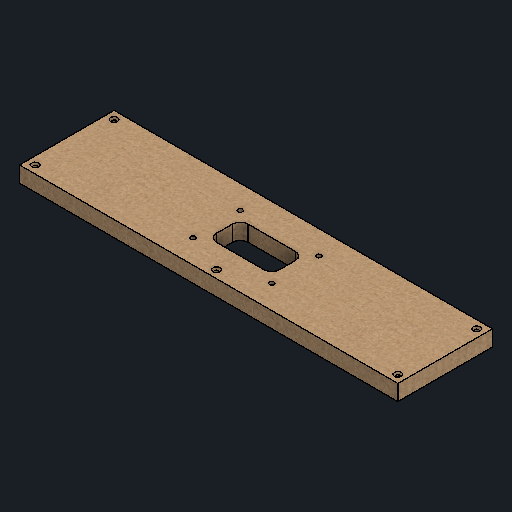
# Autodesk Inventor part: Part3
Saved by Autodesk Inventor 2026.2 (Build 302298000, 298)
## iProperties
Created: 2026-06-15
Part Number: Part3
Material: MDF Medium Density Fiberboard
Document SubType Name: Modeling
Designer: JoshuaEah
Density: 0.8 g/cm^3
Appearance: Cardboard - Corrugated
Author: JoshuaEah
Autodesk Inventor part; units mm, degrees
ref_plane "YZ Plane" through (0, 0, 0) normal (1, 0, 0) x (0, 1, 0)
ref_plane "XZ Plane" through (0, 0, 0) normal (0, 1, 0) x (-1, 0, 0)
ref_plane "XY Plane" through (0, 0, 0) normal (0, 0, 1) x (1, 0, 0)
sketch "Sketch1" plane through (0, 0, 0) normal (0, 1, 0) x (-1, 0, 0)
  line L0 (0, 0) -> (-304.8, 0)
  line L1 (-304.8, 0) -> (-304.8, -76.2)
  line L2 (-304.8, -76.2) -> (0, -76.2)
  line L3 (0, -76.2) -> (0, 0)
  line L4 (-152.4, -76.2) -> (-152.4, 0)
  line L5 (-304.8, -38.1) -> (0, -38.1)
  line L6 (-127, -50.8) -> (-177.8, -50.8)
  line L7 (-177.8, -50.8) -> (-177.8, -25.4)
  line L8 (-177.8, -25.4) -> (-127, -25.4)
  line L9 (-127, -25.4) -> (-127, -50.8)
  line L10 (-127, -50.8) -> (-177.8, -25.4) construction
  line L11 (-177.8, -50.8) -> (-127, -25.4) construction
  line L12 (-120.65, -57.15) -> (-184.15, -57.15) construction
  line L13 (-184.15, -57.15) -> (-184.15, -19.05) construction
  line L14 (-184.15, -19.05) -> (-120.65, -19.05) construction
  line L15 (-120.65, -19.05) -> (-120.65, -57.15) construction
  circle A0 centre (-120.65, -57.15) radius 1.5875
  circle A1 centre (-184.15, -57.15) radius 1.5875
  circle A2 centre (-120.65, -19.05) radius 1.5875
  circle A3 centre (-184.15, -19.05) radius 1.5875
  point P0 (-6.35, -69.85)
  point P1 (-152.4, -38.1)
  point P2 (-6.35, -69.85)
  point P3 (-298.45, -69.85)
  point P4 (-6.35, -6.35)
  point P5 (-298.45, -6.35)
  point P6 (-152.4, -6.35)
  dimension "d0" = 76.2
  dimension "d1" = 304.8
  dimension "d5" = 6.35
  dimension "d6" = 6.35
  dimension "d16" = 50.8
  dimension "d17" = 25.4
  dimension "d19" = 6.35
  dimension "d20" = 3.175
  constraints: 32 end point, 7 midpoint, 6 parallel, 6 symmetric about line, 4 centre point, 3 coincident, 3 perpendicular, 2 horizontal, 1 horizontal alignment, 1 point on line, 6 other
  measures "d0" distance of L2.end L0.start
  measures "d1" distance of L0.start L0.end
  measures "d5" distance from line of point (-6.35, -69.85) L3
  measures "d6" distance from line of L2 point (-6.35, -69.85)
  measures "d16" distance of L7.end L8.end
  measures "d17" distance of L6.end L7.end
  measures "d19" distance between parallel lines of L9 L15
  measures "d20" diameter of A0
extrude "Extrusion1" add sketch "Sketch1" against normal blind 12.7 contours L3 L5 L9 L8 L4 L0 | L4 L8 L7 L5 L1 L0 | L3 L2 L4 L6 L9 L5 | L5 L7 L6 L4 L2 L1 | A0 | A1 | A2 | A3
hole "Mounting Hole" at (6.35, 0, -69.85) direction (0, -1, 0) diameter 3.2766 end through all countersink diameter 5.715 countersink angle 82 clearance for "Flat Head Machine Screw (82)" size "#4" standard "Ansi Unified Screw Threads"
pattern_sketch "Mounting Holes" of "Mounting Hole" from (6.35, 0, -69.85) copies at (298.45, 0, -69.85) at (298.45, 0, -6.35) at (6.35, 0, -6.35) at (152.4, 0, -6.35)
sketch "Sketch2" plane through (0, 0, 0) normal (0, 1, 0) x (1, 0, 0)
  point P0 (120.65, 57.15)
  point P1 (120.65, 19.05)
  point P2 (184.15, 19.05)
  point P3 (184.15, 57.15)
hole "Jack Plate Mounting" at (120.65, 0, -57.15) direction (0, -1, 0) diameter 3.81 end through all clearance for "Flat Head Machine Screw (82)" size "#6" standard "Ansi Unified Screw Threads"
pattern_sketch "Jack Plate Mounting Holes" of "Jack Plate Mounting" from (120.65, 0, -57.15) copies at (120.65, 0, -19.05) at (184.15, 0, -19.05) at (184.15, 0, -57.15)
fillet "Fillet1" radius 6.35 4 edges at (127, -6.35, -50.8) (127, -6.35, -25.4) (177.8, -6.35, -25.4) (177.8, -6.35, -50.8)
body "Solid1"
